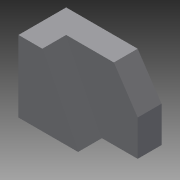
# Autodesk Inventor part: 6.7 p4
Saved by Autodesk Inventor 2015 (Build 190159000, 159)
## iProperties
Created: 2018-02-06
Part Number: 6.7 p4
Material: Generic
Document SubType Name: Modeling
Designer: Administrator
Density: 1 g/cm^3
Appearance: Default
Author: Administrator
Autodesk Inventor part; units mm, degrees
ref_plane "YZ Plane" through (0, 0, 0) normal (1, 0, 0) x (0, 1, 0)
ref_plane "XZ Plane" through (0, 0, 0) normal (0, 1, 0) x (-1, 0, 0)
ref_plane "XY Plane" through (0, 0, 0) normal (0, 0, 1) x (1, 0, 0)
sketch "Sketch1" plane through (0, 0, 0) normal (0, 0, 1) x (1, 0, 0)
  line L0 (0, 0) -> (50.8, 0)
  line L1 (38.1, 38.1) -> (0, 38.1)
  line L2 (0, 38.1) -> (0, 0)
  line L3 (50.8, 0) -> (50.8, 19.05)
  line L4 (50.8, 19.05) -> (38.1, 38.1)
  dimension "d0" = 38.1
  dimension "d1" = 50.8
  dimension "d2" = 38.1
  dimension "d3" = 19.05
  constraints: 10 end point, 1 horizontal, 1 parallel, 1 perpendicular, 1 vertical
  measures "d0" distance of L1.end L0.start
  measures "d1" distance of L0.start L0.end
  measures "d2" distance of L1.start L1.end
  measures "d3" distance of L0.end L3.end
extrude "Extrusion1" add sketch "Sketch1" along normal blind 12.7
sketch "Sketch2" plane through (0, 0, 12.7) normal (0, 0, 1) x (1, 0, 0)
  line L0 (0, 38.1) -> (0, 0)
  line L1 (0, 0) -> (31.75, 0)
  line L2 (12.7, 38.1) -> (31.75, 0)
  line L3 (12.7, 38.1) -> (0, 38.1)
  dimension "d6" = 12.7
  dimension "d7" = 31.75
  constraints: 8 end point, 1 vertical
  measures "d6" distance of L2.start L0.start
  measures "d7" distance of L0.end L1.end
extrude "Extrusion2" add sketch "Sketch2" along normal blind 12.7
body "Solid1"
